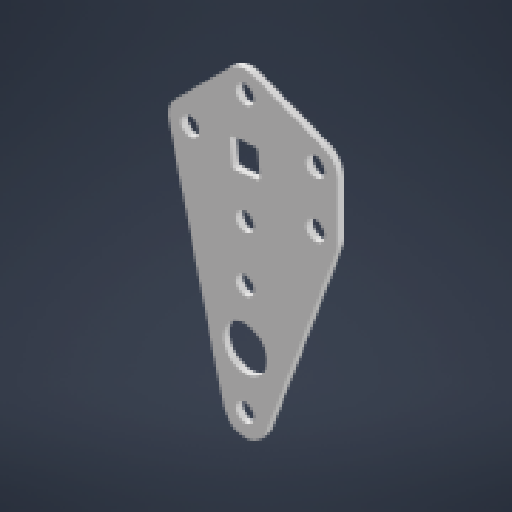
# Autodesk Inventor part: inner-pto-shaft-support
Saved by Autodesk Inventor 2023.2 (Build 272271000, 271)
## iProperties
Created: 2023-03-20
Part Number: inner-pto-shaft-support
Material: Generic
Document SubType Name: Modeling
Designer: Liam
Density: 1 g/cm^3
Appearance: Default
Author: Liam
Autodesk Inventor part; units mm, degrees
ref_plane "YZ Plane" through (0, 0, 0) normal (1, 0, 0) x (0, 1, 0)
ref_plane "XZ Plane" through (0, 0, 0) normal (0, 1, 0) x (-1, 0, 0)
ref_plane "XY Plane" through (0, 0, 0) normal (0, 0, 1) x (1, 0, 0)
sketch "Sketch1" plane through (0, 0, 0) normal (0, 0, 1) x (1, 0, 0)
  circle A0 centre (-1.1498, 6.35) radius 2.1844 projected
  circle A1 centre (-1.1498, -6.35) radius 2.1844 projected
  line L0 (-19.7028, -3.3976) -> (-14.6227, -2.9475) projected
  arc A2 (-20.3914, -2.8212) -> (-19.7028, -3.3976) centre (-19.7589, -2.7651) ccw projected
  line L1 (-20.8415, 2.2589) -> (-20.3914, -2.8212) projected
  arc A3 (-20.2651, 2.9475) -> (-20.8415, 2.2589) centre (-20.209, 2.315) ccw projected
  line L2 (-15.185, 3.3976) -> (-20.2651, 2.9475) projected
  arc A4 (-14.4964, 2.8212) -> (-15.185, 3.3976) centre (-15.1289, 2.7651) ccw projected
  line L3 (-14.0462, -2.2589) -> (-14.4964, 2.8212) projected
  arc A5 (-14.6227, -2.9475) -> (-14.0462, -2.2589) centre (-14.6788, -2.315) ccw projected
  line L4 (-17.4439, 0) -> (-17.4439, 12.7)
  circle A6 centre (-17.4439, 12.7) radius 2.1082
  circle A7 centre (-30.1439, 0) radius 2.1082
  circle A8 centre (-17.4439, -12.7) radius 2.1082
  circle A9 centre (-17.4439, -38.1) radius 5
  circle A10 centre (-17.4439, -50.8) radius 2.1082
  circle A11 centre (-17.4439, -25.4) radius 2.1082
  line L5 (-15.5993, 17.4333) -> (0.6948, 11.0833)
  line L6 (3.9302, 6.35) -> (3.9302, -6.35)
  line L7 (3.6199, -8.0984) -> (-12.6742, -52.5484)
  line L8 (-22.3722, -52.0321) -> (-35.0722, -1.2321)
  line L9 (-21.036, 16.2921) -> (-33.736, 3.5921)
  arc A12 (-15.5993, 17.4333) -> (-21.036, 16.2921) centre (-17.4439, 12.7) ccw
  arc A13 (3.9302, 6.35) -> (0.6948, 11.0833) centre (-1.1498, 6.35) ccw
  arc A14 (3.6199, -8.0984) -> (3.9302, -6.35) centre (-1.1498, -6.35) ccw
  arc A15 (-22.3722, -52.0321) -> (-12.6742, -52.5484) centre (-17.4439, -50.8) ccw
  arc A16 (-33.736, 3.5921) -> (-35.0722, -1.2321) centre (-30.1439, 0) ccw
  point P0 (0, 0)
  dimension "d11" = 12.7
  dimension "d12" = 4.2164
  dimension "d15" = 180
  dimension "d24" = 10
  dimension "d25" = 4.2164
  dimension "d26" = 4.2164
  constraints: 12 end point, 11 centre point, 10 point on circle, 4 coincident, 4 tangent, 1 vertical, 9 other
  measures "d11" distance of L4.start L4.end
  measures "d12" diameter of A6
  measures "d24" diameter of A9
  measures "d25" diameter of A11
  measures "d26" diameter of A10
extrude "Extrusion2" add sketch "Sketch1" along normal blind 1.524
body "Solid2"
